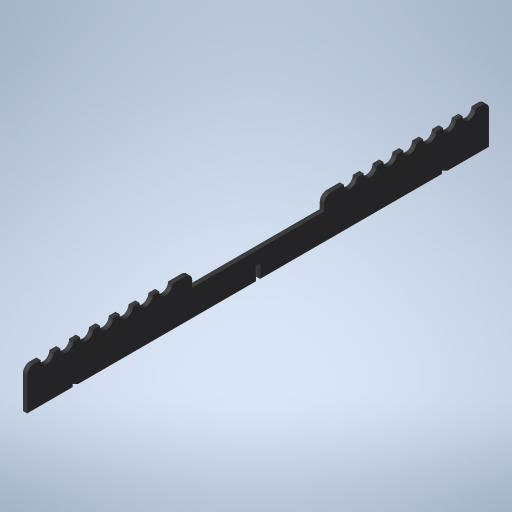
# Autodesk Inventor part: StoveTop1
Saved by Autodesk Inventor 2024.3 (Build 283343000, 343)
## iProperties
Created: 2025-06-28
Part Number: StoveTop1
Material: Generic
Document SubType Name: Modeling
Designer: ajclo
Density: 1 g/cm^3
Appearance: Default
Author: ajclo
Autodesk Inventor part; units mm, degrees
ref_plane "YZ Plane" through (0, 0, 0) normal (1, 0, 0) x (0, 1, 0)
ref_plane "XZ Plane" through (0, 0, 0) normal (0, 1, 0) x (-1, 0, 0)
ref_plane "XY Plane" through (0, 0, 0) normal (0, 0, 1) x (1, 0, 0)
sketch "Sketch1" plane through (0, 0, 0) normal (1, 0, 0) x (0, 1, 0)
  line L0 (0, 175) -> (30, 175)
  line L1 (30, 175) -> (30, -175)
  line L2 (30, -175) -> (0, -175)
  line L3 (0, -175) -> (0, 175)
  line L4 (30, 50) -> (20, 50)
  line L5 (20, 50) -> (20, -50)
  line L6 (20, -50) -> (30, -50)
  line L7 (30, -50) -> (30, 50)
  point P0 (0, 0)
  point P1 (0, 0)
  point P2 (20, 0)
  dimension "d0" = 30
  dimension "d1" = 350
  dimension "d2" = 0
  dimension "d3" = 100
  dimension "d4" = 0
  dimension "d5" = 10
  constraints: 16 end point, 4 parallel, 2 horizontal, 2 midpoint, 2 perpendicular, 1 point on line
  measures "d0" distance of L1.end L2.end
  measures "d1" distance of L0.end L1.end
  measures "d2" distance of point (0, 0) point (0, 0)
  measures "d3" distance of L4.end L5.end
  measures "d4" vertical distance of point (0, 0) point (20, 0)
  measures "d5" distance of L5.end L6.end
extrude "Extrusion1" add sketch "Sketch1" along normal blind 3 contours L0 L1 L4 L5 L6 L2 L3
sketch "Sketch2" plane through (3, 0, 0) normal (1, 0, 0) x (0, 0, -1)
  line L0 (-1.55, -10) -> (1.55, -10)
  line L1 (1.55, 0) -> (1.55, 10)
  line L2 (1.55, 10) -> (-1.55, 10)
  line L3 (-1.55, 10) -> (-1.55, 0)
  line L4 (-1.55, -10) -> (1.55, 10) construction
  line L5 (1.55, -10) -> (-1.55, 10) construction
  line L6 (-175, 0) -> (175, 0) projected
  line L7 (175, 0) -> (175, 30) projected
  line L8 (175, 30) -> (50, 30) projected
  line L9 (50, 30) -> (50, 20) projected
  line L10 (50, 20) -> (-50, 20) projected
  line L11 (-50, 20) -> (-50, 30) projected
  line L12 (-50, 30) -> (-175, 30) projected
  line L13 (-175, 30) -> (-175, 0) projected
  point P0 (0, 0)
  dimension "d8" = 3.1
  dimension "d9" = 20
  constraints: 12 end point, 2 midpoint, 2 parallel, 2 point on line, 1 horizontal, 1 perpendicular
  measures "d8" distance of L1.end L2.end
  measures "d9" distance of L0.end L1.end
extrude "Extrusion2" cut sketch "Sketch2" against normal blind 3 contours L6 L3 L2 L1
sketch "Sketch3" plane through (3, 0, 0) normal (1, 0, 0) x (0, 0, -1)
  line L0 (-50, 30) -> (-175, 30) projected
  circle A0 centre (-160, 30) radius 5
  circle A1 centre (-145, 30) radius 5
  circle A2 centre (-130, 30) radius 5
  circle A3 centre (-115, 30) radius 5
  circle A4 centre (-85, 30) radius 5
  circle A5 centre (-100, 30) radius 5
  line L1 (-175, 30) -> (-175, 0) projected
  circle A6 centre (-70, 30) radius 5
  point P0 (0, 0)
  point P1 (-75, 30)
  point P2 (-65, 30)
  point P3 (-90, 30)
  point P4 (-80, 30)
  point P5 (-105, 30)
  point P6 (-95, 30)
  point P7 (-120, 30)
  point P8 (-110, 30)
  point P9 (-135, 30)
  point P10 (-125, 30)
  point P11 (-150, 30)
  point P12 (-140, 30)
  point P13 (-165, 30)
  point P14 (-155, 30)
  dimension "d12" = 10
  dimension "d13" = 10
  dimension "d14" = 10
  dimension "d16" = 10
  dimension "d17" = 10
  dimension "d18" = 10
  dimension "d19" = 15
  dimension "d20" = 15
  dimension "d21" = 15
  dimension "d22" = 15
  dimension "d23" = 15
  dimension "d24" = 15
  dimension "d25" = 10
  dimension "d26" = 15
  constraints: 7 centre point, 5 other
  measures "d12" diameter of A0
  measures "d13" diameter of A1
  measures "d14" diameter of A2
  measures "d16" diameter of A3
  measures "d17" diameter of A4
  measures "d18" diameter of A5
  measures "d19" distance from line of L1 A0.centre
  measures "d20" distance of A1.centre A0.centre
  measures "d21" distance of A2.centre A1.centre
  measures "d22" distance of A3.centre A2.centre
  measures "d23" distance of A5.centre A3.centre
  measures "d24" distance of A5.centre A4.centre
  measures "d25" diameter of A6
  measures "d26" distance of A4.centre A6.centre
extrude "Extrusion3" cut sketch "Sketch3" against normal blind 3 contours A6 L0 | A4 L0 | A5 L0 | A3 L0 | A2 L0 | A1 L0 | A0 L0 picked at (-68.8623, 27.8538) picked at (-83.8623, 27.8538) picked at (-98.8623, 27.8538) picked at (-113.8623, 27.8538) picked at (-131.2475, 28.8948) picked at (-146.4384, 28.1203) picked at (-161.4384, 28.1203)
fillet "Fillet1" radius 5 1 edges at (1.5, 30, 175)
fillet "Fillet2" radius 5 1 edges at (1.5, 30, 50)
mirror "Mirror1" about plane through (0, 0, 0) normal (0, 0, 1) of "Extrusion3", "Fillet1", "Fillet2"
sketch "Sketch6" plane through (0, 0, 1.55) normal (0, -1, 0) x (1, 0, 0)
  line L0 (0, 0) -> (3, 0) projected
  line L1 (3, 173.45) -> (3, 0) projected
  line L2 (0, 173.45) -> (3, 173.45) projected
  line L3 (0, 173.45) -> (0, 0) projected
  line L4 (3, -3.1) -> (0, -3.1) projected
  line L5 (0, -3.1) -> (0, -176.55) projected
  line L6 (0, -176.55) -> (3, -176.55) projected
  line L7 (3, -3.1) -> (3, -176.55) projected
  line L8 (0, 142.0785) -> (3, 139.0785)
  line L9 (0, 137.8358) -> (3, 134.8358)
  line L10 (0, -137.9358) -> (3, -140.9358)
  line L11 (0, -142.1785) -> (3, -145.1785)
  line L12 (3, 0) -> (3, -3.1) projected
  line L13 (0, -1.55) -> (3, -1.55)
  point P0 (1.5, -1.55)
  dimension "d42" = 45
  dimension "d43" = 3
  dimension "d44" = 3
  dimension "d45" = 195
  dimension "d50" = 97.5
  constraints: 10 end point, 8 point on line, 3 parallel, 2 midpoint, 1 perpendicular
  measures "d42" angle of L3 L8
  measures "d43" distance between parallel lines of L9 L8
  measures "d44" distance between parallel lines of L11 L10
  measures "d45" distance between parallel lines of L10 L9
  measures "d50" distance from line of point (1.5, -1.55) L10
extrude "Extrusion5" cut sketch "Sketch6" against normal blind 2 contours L3 L8 L1 L9 | L7 L11 L5 L10
equation "\"d13\" = d12"
equation "\"d14\" = d12"
equation "\"d16\" = d12"
equation "\"d17\" = d12"
equation "\"d18\" = d12"
equation "\"d21\" = d20"
equation "\"d22\" = d21"
equation "\"d23\" = d22"
equation "\"d24\" = d23"
equation "\"d25\" = d12"
equation "\"d26\" = d24"
body "Solid1"
